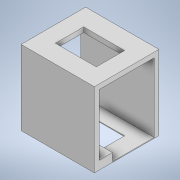
# Autodesk Inventor part: ChamberSurface
Saved by Autodesk Inventor 2022 (Build 260153000, 153)
## iProperties
Created: 2021-10-14
Part Number: ChamberSurface
Material: Generic
Document SubType Name: Modeling
Designer: iss
Density: 1 g/cm^3
Appearance: Default
Author: iss
Autodesk Inventor part; units mm, degrees
ref_plane "YZ Plane" through (0, 0, 0) normal (1, 0, 0) x (0, 1, 0)
ref_plane "XZ Plane" through (0, 0, 0) normal (0, 1, 0) x (-1, 0, 0)
ref_plane "XY Plane" through (0, 0, 0) normal (0, 0, 1) x (1, 0, 0)
sketch "Sketch1" plane through (0, 0, 0) normal (0, 1, 0) x (-1, 0, 0)
  point P0 (0, 0)
sketch "Sketch2" plane through (0, 0, 0) normal (0, 1, 0) x (-1, 0, 0)
  line L0 (23.25, -20.5) -> (-23.25, -20.5)
  line L1 (-23.25, -20.5) -> (-23.25, 20.5)
  line L2 (-23.25, 20.5) -> (23.25, 20.5)
  line L3 (23.25, 20.5) -> (23.25, -20.5)
  line L4 (23.25, -20.5) -> (-23.25, 20.5) construction
  line L5 (-23.25, -20.5) -> (23.25, 20.5) construction
  point P0 (0, 0)
  dimension "d0" = 46.5
  dimension "d1" = 41
  constraints: 12 end point, 2 midpoint, 2 parallel, 1 horizontal, 1 perpendicular
  measures "d0" distance of L1.end L2.end
  measures "d1" distance of L0.end L1.end
extrude "Extrusion1" add sketch "Sketch2" along normal blind 0.5
sketch "Sketch3" plane through (0, 0.5, 0) normal (0, 1, 0) x (1, 0, 0)
  line L0 (-13, -9) -> (13, -9)
  line L1 (13, -9) -> (13, 9)
  line L2 (13, 9) -> (-13, 9)
  line L3 (-13, 9) -> (-13, -9)
  line L4 (-13, -9) -> (13, 9) construction
  line L5 (13, -9) -> (-13, 9) construction
  point P0 (0, 0)
  dimension "d4" = 26
  dimension "d5" = 18
  constraints: 12 end point, 2 midpoint, 2 parallel, 1 horizontal, 1 perpendicular
  measures "d4" distance of L2.end L1.end
  measures "d5" distance of L1.end L0.end
extrude "Extrusion2" cut sketch "Sketch3" against normal blind 25.4
sketch "Sketch4" plane through (0, 0.5, 0) normal (0, 1, 0) x (1, 0, 0)
  line L0 (-23.25, 20.5) -> (-23.25, -20.5) projected
  line L1 (23.25, -20.5) -> (23.25, 20.5) projected
  line L2 (-23.25, -20.5) -> (23.25, -20.5)
  line L3 (23.25, -20.5) -> (23.25, -17.4625)
  line L4 (23.25, -17.4625) -> (-23.25, -17.4625)
  line L5 (-23.25, -17.4625) -> (-23.25, -20.5)
  point P0 (0, 0)
  constraints: 8 end point, 2 parallel, 1 horizontal, 1 perpendicular, 1 point on line
extrude "Extrusion3" add sketch "Sketch4" along normal blind 46.9
sketch "Sketch5" plane through (0, 0.5, 0) normal (0, 1, 0) x (1, 0, 0)
  line L0 (-23.25, 20.5) -> (-23.25, -17.4625) projected
  line L1 (-23.25, 20.5) -> (23.25, 20.5)
  line L2 (23.25, 20.5) -> (23.25, 17.4625)
  line L3 (23.25, 17.4625) -> (-23.25, 17.4625)
  line L4 (-23.25, 17.4625) -> (-23.25, 20.5)
  point P0 (0, 0)
  constraints: 8 end point, 2 parallel, 1 horizontal, 1 perpendicular
extrude "Extrusion4" add sketch "Sketch5" along normal blind 46.9
sketch "Sketch6" plane through (23.25, 0.5, 17.4625) normal (0, 0, -1) x (-1, 0, 0)
  point P0 (23.25, -0.5)
sketch "Sketch7" plane through (23.25, 0.5, 17.4625) normal (0, 0, -1) x (-1, 0, 0)
  point P0 (23.25, -0.5)
sketch "Sketch8" plane through (23.25, 0.5, 17.4625) normal (0, 0, -1) x (-1, 0, 0)
  line L0 (46.5, 0) -> (46.5, 46.9) projected
  line L1 (0, 0) -> (0, 46.9) projected
  line L2 (46.5, 46.9) -> (0, 46.9)
  line L3 (0, 46.9) -> (0, 43.8105)
  line L4 (0, 43.8105) -> (46.5, 43.8105)
  line L5 (46.5, 43.8105) -> (46.5, 46.9)
  point P0 (23.25, -0.5)
  constraints: 8 end point, 2 parallel, 1 horizontal, 1 perpendicular, 1 point on line
extrude "Extrusion5" add sketch "Sketch8" along normal blind 35
sketch "Sketch9" plane through (0, 47.4, 0) normal (0, 1, 0) x (1, 0, 0)
  line L0 (-13, -9) -> (-13, 9) projected
  line L1 (13, 9) -> (-13, 9)
  line L2 (-13, 9) -> (-13, -9)
  line L3 (-13, -9) -> (13, -9)
  line L4 (13, -9) -> (13, 9)
  line L5 (13, 9) -> (-13, -9) construction
  line L6 (-13, 9) -> (13, -9) construction
  point P0 (0, 0)
  constraints: 12 end point, 2 midpoint, 2 parallel, 1 horizontal, 1 perpendicular
sketch "Sketch10" plane through (0, 0.5, 0) normal (0, 1, 0) x (1, 0, 0)
  point P0 (0, 0)
sketch "Sketch11" plane through (0, 0.5, 0) normal (0, 1, 0) x (1, 0, 0)
  line L0 (-23.25, -17.4625) -> (23.25, -17.4625) projected
  line L1 (-23.25, -17.4625) -> (-18.283, -17.4625)
  line L2 (-18.283, -17.4625) -> (-18.283, 17.4625)
  line L3 (-18.283, 17.4625) -> (-23.25, 17.4625)
  line L4 (-23.25, 17.4625) -> (-23.25, -17.4625)
  point P0 (0, 0)
  constraints: 8 end point, 2 parallel, 1 horizontal, 1 perpendicular
extrude "Extrusion6" add sketch "Sketch11" along normal blind 2.9718
extrude "Extrusion7" cut sketch "Sketch9" against normal blind 4.9657
sketch "Sketch12" plane through (0, 0.5, 0) normal (0, 1, 0) x (1, 0, 0)
  point P0 (0, 0)
sketch "Sketch13" plane through (0, 0.5, 0) normal (0, 1, 0) x (1, 0, 0)
  line L0 (23.25, -17.4625) -> (23.25, 17.4625) projected
  line L1 (-14.2875, -17.4625) -> (23.25, -17.4625)
  line L2 (23.25, -17.4625) -> (23.25, -9.0284)
  line L3 (23.25, -9.0284) -> (-14.2875, -9.0284)
  line L4 (-14.2875, -9.0284) -> (-14.2875, -17.4625)
  point P0 (0, 0)
  constraints: 8 end point, 2 parallel, 1 horizontal, 1 perpendicular, 1 point on line
extrude "Extrusion8" add sketch "Sketch13" along normal blind 4.9657
body "Solid1"
